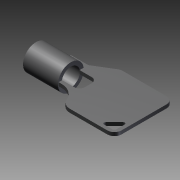
# Autodesk Inventor part: LOCNL2_k
Saved by Autodesk Inventor 2011 SP1 (Build 150282100, 282)
## iProperties
Created: 2015-03-21
Part Number: LOCNL2_k
Catalog Web Link: www.cadenas.de
Description: LOCNL_k-Knuckle Locks
Vendor: MISUMI
Document SubType Name: Modeling
Designer: PARTuser1
Manufacturer: MISUMI
Mass: 0.514905 g
Surface Area: 11.2498 cm^2
Volume: 0.514905 cm^3
Density: 1 g/cm^3
Category: PARTsolutions
Company: MISUMI
Title: LOCNL2_k
Author: Cadenas PARTsolutions
Comments: Knuckle Locks
PSOL_IDENT_0: {\\10.0.0.236\data_v8\23d-libs\misumi\metric\44_handles_hinges\locnl_k.prj},159 {VTYP=3D},{NB=LOCNL2
PSOL_IDENT_1: _k},{LINA=LOCNL2_k},{NN=LOCNL_k},{DATE=14.11.2014 09:15:19},{GEOMDATE=09.12.2008 13:39:00},{VERSION=
PSOL_IDENT_2: },{LINEID=20},{LINESUBID=-1},{WBVAR=}  {NB=LOCNL2_k},{LINA=LOCNL2_k},{KT=DUMMY},{PN=LOCNL2},{TYPE=LO
PSOL_IDENT_3: CNL},{MATMB=Zinc Die Casting},{MATHN=Low Carbon Steel},{MATLP=Low Carbon Steel},{MATK=Low Carbon Ste
PSOL_IDENT_4: el},{STMB=Chrome Plating},{STHN=Trivalent Chromate},{STLP=Trivalent Chromate},{STK=Chrome Plating},{
PSOL_IDENT_5: NO=2},{KD=2  Holes},{MASS=25},{AK=2 Pcs.}
SUPPLIER: MISUMI
ARTICLENO: LOCNL2_k
BOMINFO: LOCNL2_k
CREATOR: CADENAS GmbH
Autodesk Inventor part; units mm, degrees
sketch "Sketch_1" plane through (0, 0, 0) normal (1, 0, 0) x (0, 1, 0)
  circle A0 centre (0, 0) radius 3.707
  circle A1 centre (0, 0) radius 2.607
  constraints: 2 centre point
extrude "Extrusion1" add sketch "Sketch_1" along normal blind 10
sketch "Sketch_2" plane through (0, 0, 0) normal (1, 0, 0) x (0, 1, 0)
  line L0 (2.0509, 0.55) -> (2.0509, -0.55)
  line L1 (2.0509, -0.55) -> (4.6009, -0.55)
  line L2 (4.6009, -0.55) -> (4.6009, 0.55)
  line L3 (4.6009, 0.55) -> (2.0509, 0.55)
  constraints: 8 end point
extrude "Extrusion2" add sketch "Sketch_2" along normal blind 0.5
sketch "Sketch_3" plane through (0, 0, 0) normal (1, 0, 0) x (0, 1, 0)
  line L0 (0.55, -2.0509) -> (-0.55, -2.0509)
  line L1 (-0.55, -2.0509) -> (-0.55, -4.6009)
  line L2 (-0.55, -4.6009) -> (0.55, -4.6009)
  line L3 (0.55, -4.6009) -> (0.55, -2.0509)
  constraints: 8 end point
extrude "Extrusion3" add sketch "Sketch_3" along normal blind 0.5
sketch "Sketch_4" plane through (0, 0, 0) normal (0, 0, 1) x (1, 0, 0)
  line L0 (5, 5) -> (5, 3.5)
  line L1 (5, 3.5) -> (10, 3.5)
  line L2 (10, 3.5) -> (10, 2.5)
  line L3 (10, 2.5) -> (13.5, 2.5)
  arc A0 (15, 1) -> (13.5, 2.5) centre (13.5, 1) ccw
  line L4 (15, 1) -> (15, -1)
  arc A1 (13.5, -2.5) -> (15, -1) centre (13.5, -1) ccw
  line L5 (13.5, -2.5) -> (10, -2.5)
  line L6 (10, -2.5) -> (10, -3.5)
  line L7 (10, -3.5) -> (10.7881, -3.5)
  arc A2 (15.4232, -6.625) -> (10.7881, -3.5) centre (10.7881, -8.5) ccw
  arc A3 (15.4232, -6.625) -> (18.2043, -8.5) centre (18.2043, -5.5) ccw
  line L8 (18.2043, -8.5) -> (29, -8.5)
  arc A4 (29, -8.5) -> (31, -6.5) centre (29, -6.5) ccw
  line L9 (31, -6.5) -> (31, 6.5)
  arc A5 (31, 6.5) -> (29, 8.5) centre (29, 6.5) ccw
  line L10 (29, 8.5) -> (16.3458, 8.5)
  arc A6 (16.3458, 8.5) -> (15.3109, 8.2114) centre (16.3458, 6.5) ccw
  line L11 (15.3109, 8.2114) -> (10.1193, 5.0721)
  arc A7 (9.8606, 5) -> (10.1193, 5.0721) centre (9.8606, 5.5) ccw
  line L12 (9.8606, 5) -> (5, 5)
  arc A8 (26.7036, -6.6464) -> (27.0571, -7.5) centre (27.0571, -7) ccw
  line L13 (27.0571, -7.5) -> (29.5, -7.5)
  arc A9 (29.5, -7.5) -> (30, -7) centre (29.5, -7) ccw
  line L14 (30, -7) -> (30, -4.5571)
  arc A10 (30, -4.5571) -> (29.1464, -4.2036) centre (29.5, -4.5571) ccw
  line L15 (29.1464, -4.2036) -> (26.7036, -6.6464)
  constraints: 32 end point, 22 point on circle, 11 centre point
extrude "Extrusion4" add sketch "Sketch_4" along normal mid plane 1
ref_plane "k_to_1_XY" through (0, 0, 0) normal (1, 0, 0) x (0, 0, -1)
ref_plane "k_to_1_YZ" through (0, 0, 0) normal (0, 0, -1) x (0, 1, 0)
ref_plane "k_to_1_ZX" through (0, 0, 0) normal (0, 1, 0) x (1, 0, 0)
ref_plane "3_TO_K_XY" through (27, -6.5, 0) normal (0, 0, 1) x (1, 0, 0)
ref_plane "3_TO_K_YZ" through (27, -6.5, 0) normal (1, 0, 0) x (0, 1, 0)
ref_plane "3_TO_K_ZX" through (27, -6.5, 0) normal (0, 1, 0) x (0, 0, 1)
ref_plane "K1_TO_3_XY" through (29, -3, 0) normal (1, 0, 0) x (0, 0, -1)
ref_plane "K1_TO_3_YZ" through (29, -3, 0) normal (0, 0, -1) x (0, 1, 0)
ref_plane "K1_TO_3_ZX" through (29, -3, 0) normal (0, 1, 0) x (1, 0, 0)
body "Solid1"
